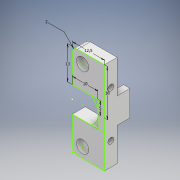
# Autodesk Inventor part: togh
Saved by Autodesk Inventor 2018 (Build 220112000, 112)
## iProperties
Created: 2017-05-26
Part Number: togh
Material: ABS Plastic
Document SubType Name: Modeling
Designer: Karol
Density: 1.06 g/cm^3
Appearance: Smooth - White
Author: Karol
Autodesk Inventor part; units mm, degrees
ref_plane "YZ Plane" through (0, 0, 0) normal (1, 0, 0) x (0, 1, 0)
ref_plane "XZ Plane" through (0, 0, 0) normal (0, 1, 0) x (-1, 0, 0)
ref_plane "XY Plane" through (0, 0, 0) normal (0, 0, 1) x (1, 0, 0)
sketch "Sketch1" plane through (0, 0, 0) normal (0, 1, 0) x (-1, 0, 0)
  line L0 (-3.25, 0) -> (-3.25, 5)
  line L1 (-3.25, 5) -> (6.75, 5)
  line L2 (6.75, 5) -> (6.75, 16)
  arc A0 (-0.5666, 5) -> (-3.25, 0) centre (2.75, 0) ccw
  line L3 (-5.75, 0) -> (-5.75, 18)
  line L4 (-5.75, 18) -> (4.75, 18)
  arc A1 (6.75, 16) -> (4.75, 18) centre (4.75, 16) ccw
  line L5 (-3.25, 0) -> (-3.25, -5)
  line L6 (-3.25, -5) -> (6.75, -5)
  line L7 (6.75, -5) -> (6.75, -16)
  arc A2 (-3.25, 0) -> (-0.5666, -5) centre (2.75, 0) ccw
  line L8 (-5.75, 0) -> (-5.75, -18)
  line L9 (-5.75, -18) -> (4.75, -18)
  arc A3 (4.75, -18) -> (6.75, -16) centre (4.75, -16) ccw
  line L10 (-3.25, -5) -> (-5.75, -5)
  line L11 (-3.25, 5) -> (-5.75, 5)
  point P0 (2.75, 14)
  point P1 (6.75, 18)
  point P2 (6.75, 18)
  point P3 (2.75, -14)
  point P4 (6.75, -18)
  point P5 (6.75, -18)
  dimension "d29" = 5
  dimension "d32" = 10
  dimension "d68" = 13
  dimension "d69" = 18
  dimension "d70" = 12.5
  dimension "d71" = 2
  constraints: 24 end point, 8 point on circle, 8 point on line, 4 centre point, 3 vertical, 2 horizontal, 2 perpendicular, 2 tangent
  measures "d29" distance of L0.start L0.end
  measures "d32" distance of L0.end L1.end
  measures "d68" distance of L1.end point (6.75, 18)
  measures "d69" distance of L3.start L3.end
  measures "d70" distance of L3.end point (6.75, 18)
  measures "d71" radius of A1
extrude "Extrusion1" add sketch "Sketch1" along normal blind 5 contours L5 L10 L8 L3 L11 L0 | L11 L3 L4 A1 L2 L1 | L6 L7 A3 L9 L8 L10
sketch "Sketch5" plane through (-6.75, 0, 5) normal (-1, 0, 0) x (0, 0, 1)
  point P0 (-5, 0)
  point P1 (4, 2.5)
  point P2 (-14, 2.5)
hole "Hole3" at (-6.75, 2.5, 9) at (-6.75, 2.5, -9) direction (1, 0, 0) diameter 2.3 depth 13
hole "Hole5" at (-2.75, 0, 14) at (-2.75, 0, -14) direction (0, 1, 0) diameter 4.8 depth 8 tip angle 118
extrude "Extrusion8" add sketch "Sketch1" along normal blind 10 contours L5 L10 L8 L3 L11 L0
body "Solid1"
